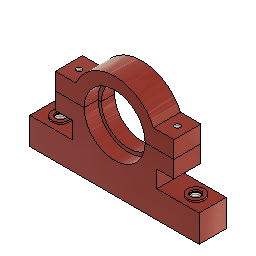
MANCAL v1 (Autodesk Fusion 360 design; units mm, degrees)
Autodesk Fusion 360 part; units mm, degrees
sketch "Esboço1" plane through (0, 0, 0) normal (0, 1, 0) x (1, 0, 0)
  circle A0 centre (0, 0) radius 8
  circle A1 centre (0, 0) radius 9
  circle A2 centre (0, 0) radius 12.5
  line L0 (-25.0547, 18) -> (24.9453, 18)
  line L1 (24.9453, 18) -> (24.9453, 10)
  line L2 (24.9453, 10) -> (7.5, 10)
  line L3 (-7.5, 10) -> (-25.0547, 10)
  line L4 (-25.0547, 10) -> (-25.0547, 18)
  line L5 (-12.5, 0) -> (-12.5, 10)
  line L6 (12.5, 0) -> (12.5, 10)
  line L7 (-0.0547, -12.4999) -> (-0.0547, 18) construction
  line L8 (12.5, 0) -> (-12.5, 0)
  dimension "d1" = 16
  dimension "d2" = 18
  dimension "d3" = 25
  dimension "d5" = 25
  dimension "d7" = 25
  dimension "d76" = 10
  dimension "d77" = 10
  dimension "d78" = 8
  constraint coincident A0.centre A1.centre
  constraint concentric A0 A1
  constraint concentric A1 A2
  constraint horizontal L0
  constraint perpendicular L0 L1
  constraint coincident A2 L2.end
  constraint perpendicular L1 L2
  constraint coincident A2 L3.start
  constraint perpendicular L1 L3
  constraint perpendicular L0 L4
  constraint coincident A2 L5.start
  constraint coincident L3 L5.end
  constraint perpendicular L3 L5
  constraint coincident A2 L6.start
  constraint coincident L2 L6.end
  constraint tangent A2 L6
  constraint perpendicular L2 L6
  constraint coincident A2 L7.start
  constraint coincident L0 L7.end
  constraint perpendicular L0 L7
  constraint perpendicular L5 L8
  measures "d1" diameter of A0
  measures "d2" diameter of A1
  measures "d3" diameter of A2
  measures "d5" distance of L1 L7
  measures "d7" distance of L4 L7
  measures "d76" distance of L5.start L5.end
  measures "d77" distance of L6.start L6.end
  measures "d78" distance of L0.end L1.end
extrude "Extrusão1" add sketch "Esboço1" along normal blind 8 contours A0 A1 L8 | A0 A1 L8 | A1 A2 L8 | A1 A2 L8 | A2 L2 L6 | A2 L3 L5 | A2 L0 L1 L2 L3 L4 makes body 1
extrude "Extrusão2" cut sketch "Esboço1" along normal blind 4.1 contours A0 A1 L8 | A0 A1 L8 bodies 1
sketch "Esboço2" plane through (0, 0, -10) normal (0, 0, 1) x (-1, 0, 0)
  line L0 (25.0547, 0) -> (12.5, 0)
  line L1 (12.5, 0) -> (12.5, -8)
  line L2 (12.5, -8) -> (25.0547, -8)
  line L3 (25.0547, -8) -> (25.0547, 0)
  circle A0 centre (20, -4) radius 1.5
  circle A1 centre (-20, -4) radius 1.5
  circle A2 centre (20, -4) radius 2.5
  circle A3 centre (-20, -4) radius 2.5
  line L4 (25.0547, -4) -> (-25, -4) construction
  line L5 (0, -10) -> (0, 3) construction
  dimension "d12" = 3
  dimension "d13" = 3
  dimension "d18" = 5
  dimension "d19" = 5
  dimension "d74" = 20
  dimension "d75" = 20
  constraint concentric A0 A2
  constraint concentric A1 A3
  constraint midpoint L3 L4.start
  constraint perpendicular L3 L4
  constraint coincident A0.centre L4
  constraint coincident A1.centre L4
  constraint vertical L5
  measures "d12" diameter of A0
  measures "d13" diameter of A1
  measures "d18" diameter of A2
  measures "d19" diameter of A3
  measures "d74" distance of A1.centre L5
  measures "d75" distance of A0.centre L5
extrude "Extrusão3" cut sketch "Esboço2" against normal blind 8 contours A0 | A1 bodies 1
thread "Rosca1" "ISO Metric profile 3.0 M3x0.5 M3x0.5 6H" major diameter 3.086 minor diameter 2.529 pitch 0.5 angle 60 resizes the face on face at (-21.4925, 4.1494, -15.3333) on face at (18.5075, 4.1494, -15.3333) on bodies 1
extrude "Extrusão4" add sketch "Esboço2" along normal blind 0.5 contours A2 | A3 bodies 1
extrude "Extrusão5" cut sketch "Esboço1" along normal blind 21 contours A0 A1 L8 | A0 L8 | A1 A2 L8 picked at (-8.6332, -0.4471) picked at (2.0435, -5.9488) picked at (-11.2868, -0.621) bodies 1
sketch "Esboço1 (2)" plane through (0, 0, 0) normal (0, 1, 0) x (1, 0, 0) in component "PARTE DE CIMA"
  line L0 (19.9453, 15) -> (19.9453, 10)
  line L1 (-20.0547, 15) -> (19.9453, 15)
  line L2 (12.5, 0) -> (-12.5, 0)
  circle A0 centre (0, 0) radius 8
  line L3 (-20.0547, 10) -> (-20.0547, 15)
  line L4 (-7.5, 10) -> (-20.0547, 10)
  line L5 (12.5, 0) -> (12.5, 10)
  circle A1 centre (0, 0) radius 9
  line L6 (-0.0547, -12.4999) -> (-0.0547, 15) construction
  circle A2 centre (0, 0) radius 12.5
  line L7 (19.9453, 10) -> (7.5, 10)
  line L8 (-12.5, 0) -> (-12.5, 10)
  line L9 (-11.4379, -5.0423) -> (-17.4999, -5.0423)
  line L10 (-17.4999, -5.0423) -> (-17.4999, 0)
  line L11 (-17.4999, 0) -> (-12.5, 0)
  line L12 (11.4379, -5.0423) -> (17.4999, -5.0423)
  line L13 (17.4999, -5.0423) -> (17.4999, 0)
  line L14 (17.4999, 0) -> (12.5, 0)
  dimension "d24" = 16
  dimension "d25" = 18
  dimension "d26" = 25
  dimension "d27" = 20
  dimension "d28" = 20
  dimension "d52" = 6.062
  dimension "d53" = 6.062
  constraint coincident A0.centre A1.centre
  constraint concentric A0 A1
  constraint concentric A1 A2
  constraint horizontal L1
  constraint perpendicular L0 L1
  constraint coincident L7.end A2
  constraint perpendicular L0 L7
  constraint coincident L4.start A2
  constraint perpendicular L0 L4
  constraint perpendicular L1 L3
  constraint coincident L2.end A2
  constraint coincident L8.end L4
  constraint perpendicular L4 L8
  constraint coincident L2.start A2
  constraint coincident L5.end L7
  constraint tangent L5 A2
  constraint perpendicular L5 L7
  constraint coincident L6.start A2
  constraint coincident L6.end L1
  constraint perpendicular L1 L6
  constraint perpendicular L2 L8
  constraint coincident A2 L9.start
  constraint horizontal L9
  constraint perpendicular L9 L10
  constraint perpendicular L8 L11
  constraint coincident A2 L12.start
  constraint parallel L11 L12
  constraint perpendicular L12 L13
  constraint perpendicular L5 L14
  measures "d24" diameter of A0
  measures "d25" diameter of A1
  measures "d26" diameter of A2
  measures "d27" distance of L0 L6
  measures "d28" distance of L3 L6
  measures "d52" distance of L9.start L9.end
  measures "d53" distance of L12.start L12.end
extrude "Extrusão1'" add sketch "Esboço1 (2)" along normal blind 8 separate body contours L2 A1 A2 | A2 L12 L13 L14 | L2 A0 A1 | A2 L9 L10 L11 picked at (-0.824, -11.2816) picked at (-8.6332, -0.4471) makes body 2 in component "Component"
sketch "Esboço2 (2)" plane through (0, 0, 5.0423) normal (0, 0, 1) x (-1, 0, 0) in component "PARTE DE CIMA"
  line L0 (-11.4379, 0) -> (-17.4999, 0)
  line L1 (-17.4999, 0) -> (-17.4999, -8)
  line L2 (-17.4999, -8) -> (-11.4379, -8)
  line L3 (-11.4379, -8) -> (-11.4379, 0)
  circle A0 centre (13.3, -4.0301) radius 1
  circle A1 centre (-13.3, -4.0301) radius 1
  line L4 (0, -8) -> (0, 0) construction
  dimension "d31" = 2
  dimension "d32" = 2
  dimension "d33" = 13.3
  dimension "d34" = 13.3
  constraint coincident L4.end origin
  constraint parallel L3 L4
  measures "d31" diameter of A0
  measures "d32" diameter of A1
  measures "d33" distance of A0.centre L4
  measures "d34" distance of A1.centre L4
extrude "Extrusão1''" [suppressed] in component "PARTE DE CIMA"
extrude "Extrusão3'" cut sketch "Esboço1 (2)" along normal blind 4.1 contours L2 A0 A1 picked at (-8.6332, -0.4471) bodies 2 in component "Component"
sketch "Esboço3" plane through (0, 0, 0) normal (0, 1, 0) x (1, 0, 0)
  line L0 (-17.4999, -5.0423) -> (-17.4999, 0)
  line L1 (-11.4379, -5.0423) -> (-17.4999, -5.0423)
  line L2 (12.5, 0) -> (12.5, 10)
  line L3 (-12.5, 0) -> (-12.5, 10)
  line L4 (-17.4999, 0) -> (-12.5, 0)
  line L5 (15, 0) -> (12.5, 0)
  line L6 (-17.5, 5) -> (-17.5, 0)
  line L7 (-17.5, 0) -> (-17.4999, 0)
  line L8 (-17.5, 5) -> (-12.5, 5)
  line L9 (0, -13) -> (0, 15) construction
  line L10 (17.5, 0) -> (17.4999, 0)
  line L11 (17.5, 5) -> (17.5, 0)
  line L12 (17.5, 5) -> (12.5, 5)
  line L13 (17.4999, 0) -> (12.5, 0)
  dimension "d41" = 5.0423
  dimension "d42" = 6.062
  dimension "d51" = 5
  constraint coincident L0.end L4.start
  constraint coincident L3.start L4.end
  constraint coincident L2.start L5.end
  constraint perpendicular L2 L5
  constraint perpendicular L0 L7
  constraint midpoint L3 L8.end
  constraint perpendicular L3 L8
  constraint vertical L9
  constraint symmetric L6.start L9 L11.start
  constraint symmetric L0.end L9 L10.end
  constraint symmetric L3.start L9 L2.start
  constraint symmetric L6.end L9 L10.start
  constraint symmetric L8.end L9 L12.end
  measures "d41" distance of L0.start L0.end
  measures "d42" distance of L0.start L1.start
  measures "d51" distance of L6.start L8.end
extrude "Extrusão6" add sketch "Esboço3" along normal blind 8 bodies 1
sketch "Esboço5" plane through (0, 0, 0) normal (0, 0, 1) x (-1, 0, 0)
  line L0 (8, -8) -> (17.5, -8)
  line L1 (17.5, -8) -> (17.5, 0)
  line L2 (17.5, 0) -> (9, 0)
  line L3 (9, 0) -> (9, -4.1)
  line L4 (9, -4.1) -> (8, -4.1)
  line L5 (8, -4.1) -> (8, -8)
  line L6 (0, -10) -> (0, 1) construction
  circle A0 centre (14.5, -4) radius 1
  circle A1 centre (-14.5, -4) radius 1
  dimension "d58" = 2
  dimension "d59" = 2
  dimension "d60" = 14.5
  dimension "d61" = 14.5
  constraint vertical L6
  measures "d58" diameter of A0
  measures "d59" diameter of A1
  measures "d60" distance of L6 A0.centre
  measures "d61" distance of L6 A1.centre
extrude "Extrusão8" cut sketch "Esboço5" against normal blind 5 contours A0 | A1 bodies 1
thread "Rosca2" "ISO Metric profile 2.0 M2x0.4 M2x0.4 6H" major diameter 2.074 minor diameter 1.623 pitch 0.4 angle 60 resizes the face on face at (-15.4988, 4.0498, -3.3333) on face at (13.5012, 4.0498, -3.3333) on bodies 1
sketch "Esboço3 (2)" plane through (0, 0, 5.0423) normal (0, 0, 1) x (-1, 0, 0) in component "PARTE DE CIMA"
  line L0 (17.4999, 0) -> (11.4379, 0)
  line L1 (11.4379, 0) -> (11.4379, -8)
  line L2 (11.4379, -8) -> (17.4999, -8)
  line L3 (17.4999, -8) -> (17.4999, 0)
  circle A0 centre (14.5, -4) radius 1
  circle A1 centre (-14.5, -4) radius 1
  line L4 (0, -9) -> (0, 1.4718) construction
  dimension "d66" = 2
  dimension "d67" = 2
  dimension "d68" = 14.5
  dimension "d69" = 14.5
  constraint vertical L4
  measures "d66" diameter of A1
  measures "d67" diameter of A0
  measures "d68" distance of A0.centre L4
  measures "d69" distance of A1.centre L4
extrude "Extrusão5'" cut sketch "Esboço3 (2)" against normal blind 6 contours A0 | A1 bodies 2 in component "Component"
thread "Rosca1'" "ISO Metric profile 2.0 M2x0.4 M2x0.4 6H" major diameter 2.074 minor diameter 1.623 pitch 0.4 angle 60 resizes the face on face at (13.505, 4.0996, 3.3616) on face at (-15.495, 4.0996, 3.3616) on bodies 2 in component "Component"
component "PARTE DE CIMA" placed x (1, 0, 0) y (0, 1, 0) z (0, 0, 1) at (0, 0, 0)
component "Component" placed x (1, 0, 0) y (0, 1, 0) z (0, 0, 1) at (0, 0, 0) in component "PARTE DE CIMA"
